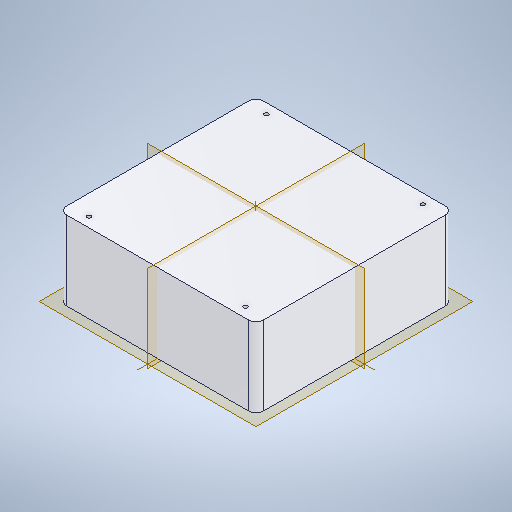
# Autodesk Inventor part: BOX
Saved by Autodesk Inventor 2025.2 (Build 292293000, 293)
## iProperties
Created: 2025-04-12
Part Number: BOX
Material: Generic
Document SubType Name: Modeling
Designer: yehorderehus
Density: 1 g/cm^3
Appearance: PTFE
Author: yehorderehus
Autodesk Inventor part; units mm, degrees
sketch "Sketch1" plane through (0, 0, 0) normal (0, 1, 0) x (-1, 0, 0)
  line L0 (-75, 75) -> (75, 75)
  line L1 (75, 75) -> (75, -75)
  line L2 (75, -75) -> (-75, -75)
  line L3 (-75, -75) -> (-75, 75)
  line L4 (-75, 75) -> (75, -75) construction
  line L5 (75, 75) -> (-75, -75) construction
  point P0 (0, 0)
  dimension "d0" = 150
  dimension "d1" = 150
  constraints: 12 end point, 2 midpoint, 2 parallel, 1 horizontal, 1 perpendicular
  measures "d0" distance of L1.end L2.end
  measures "d1" distance of L2.end L0.start
extrude "Extrusion1" add sketch "Sketch1" along normal blind 60
sketch "Sketch2" plane through (0, 60, 0) normal (0, 1, 0) x (1, 0, 0)
  circle A0 centre (-59.5, 67.5) radius 1.5
  circle A1 centre (59.5, 67.5) radius 1.5
  circle A2 centre (59.5, -67.5) radius 1.5
  circle A3 centre (-59.5, -67.5) radius 1.5
  line L0 (0, 105) -> (0, -105) projected
  line L1 (105, 0) -> (-105, 0) projected
  circle A4 centre (-59.5, 67.5) radius 1.5
  circle A5 centre (59.5, 67.5) radius 1.5
  circle A6 centre (59.5, -67.5) radius 1.5
  circle A7 centre (-59.5, -67.5) radius 1.5
  point P0 (0, 0)
  dimension "d4" = 3
  dimension "d5" = 119
  dimension "d6" = 135
  dimension "d7" = 59.5
  dimension "d8" = 67.5
  dimension "d11" = 3
  constraints: 8 centre point, 6 equal radius, 4 coincident, 2 horizontal alignment, 2 vertical alignment
  measures "d4" diameter of A0
  measures "d5" distance of A1.centre A0.centre
  measures "d6" distance of A2.centre A1.centre
  measures "d7" distance from line of A0.centre L0
  measures "d8" distance from line of L1 A0.centre
  measures "d11" diameter of A4
extrude "Extrusion2" cut sketch "Sketch2" against normal through all
fillet "Fillet1" radius 6 4 edges at (75, 30, 75) (-75, 30, 75) (75, 30, -75) (-75, 30, -75)
equation "\"d7\" = 0.5 * d5"
equation "\"d8\" = 0.5 * d6"
body "Solid1"
